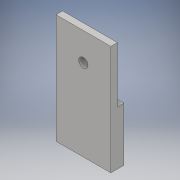
# Autodesk Inventor part: Metal_mount_vertical_v1
Saved by Autodesk Inventor 2017 (Build 210142000, 142)
## iProperties
Created: 2019-10-14
Part Number: Metal_mount_vertical_v1
Material: Generic
Document SubType Name: Modeling
Designer: nvladim
Density: 1 g/cm^3
Appearance: Default
Author: nvladim
Autodesk Inventor part; units mm, degrees
ref_plane "YZ Plane" through (0, 0, 0) normal (1, 0, 0) x (0, 1, 0)
ref_plane "XZ Plane" through (0, 0, 0) normal (0, 1, 0) x (-1, 0, 0)
ref_plane "XY Plane" through (0, 0, 0) normal (0, 0, 1) x (1, 0, 0)
sketch "Sketch1" plane through (0, 0, 0) normal (0, 1, 0) x (-1, 0, 0)
  line L0 (0, 0) -> (24.6, 0)
  line L1 (50, 0) -> (50, -25)
  line L2 (50, -25) -> (24.6, -25)
  line L3 (0, -25) -> (0, 0)
  line L4 (50, 0) -> (24.6, 0) construction
  line L5 (24.6, 0) -> (24.6, -25)
  line L6 (24.6, -25) -> (50, -25) construction
  line L7 (50, -25) -> (50, 0) construction
  line L8 (24.6, 0) -> (50, 0)
  line L9 (24.6, -25) -> (0, -25)
  point P0 (37.3, -12.5)
  dimension "d0" = 50
  dimension "d1" = 25
  dimension "d2" = 25.4
  constraints: 20 end point, 7 parallel, 3 horizontal, 3 perpendicular
  measures "d0" distance of L1.end L3.start
  measures "d1" distance of L1.start L1.end
  measures "d2" distance of L6.end L2.end
extrude "Extrusion1" add sketch "Sketch1" along normal blind 3 contours L8 L1 L2 L5
hole "Hole1" at (-37.3, 0, -12.5) direction (0, 1, 0) diameter 4.2 end through all
extrude "Extrusion2" add sketch "Sketch1" along normal blind 3 contours L0 L5 L9 L3
extrude "Extrusion3" add sketch "Sketch1" against normal blind 3 contours L0 L5 L9 L3
sketch "Sketch2" plane through (0, 3, 0) normal (1, 0, 0) x (0, 0, -1)
  line L0 (12.5, -0.947) -> (12.5, -4.9651)
  line L1 (25, -3) -> (0, -3) projected
  point P0 (6.25, -3)
  point P1 (18.75, -3)
  constraints: 2 end point, 1 point on line, 1 symmetric about line, 1 vertical
hole "Hole2" at (0, 0, -18.75) at (0, 0, -6.25) direction (-1, 0, 0) diameter 2.5 depth 10 tip angle 118
body "Solid1"
